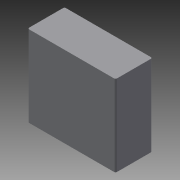
# Autodesk Inventor part: Battery(Raw)
Saved by Autodesk Inventor 2014 SP1 (Build 180222100, 222)
## iProperties
Created: 2014-03-26
Part Number: Battery(Raw)
Material: Generic
Document SubType Name: Modeling
Designer: carpenma
Density: 1 g/cm^3
Appearance: Default
Author: carpenma
Autodesk Inventor part; units mm, degrees
ref_plane "YZ Plane" through (0, 0, 0) normal (1, 0, 0) x (0, 1, 0)
ref_plane "XZ Plane" through (0, 0, 0) normal (0, 1, 0) x (-1, 0, 0)
ref_plane "XY Plane" through (0, 0, 0) normal (0, 0, 1) x (1, 0, 0)
sketch "Sketch1" plane through (0, 0, 0) normal (0, 0, 1) x (1, 0, 0)
  line L0 (0, 0) -> (181.102, 0)
  line L1 (181.102, 0) -> (181.102, 166.878)
  line L2 (181.102, 166.878) -> (0, 166.878)
  line L3 (0, 166.878) -> (0, 0)
  dimension "d0" = 181.102
  dimension "d1" = 166.878
  constraints: 8 end point, 2 parallel, 1 horizontal, 1 perpendicular
  measures "d0" distance of L2.end L1.end
  measures "d1" distance of L1.end L0.end
extrude "Extrusion1" add sketch "Sketch1" against normal blind 75.946
fillet "Fillet1" radius 3.175 4 edges at (0, 83.439, 0) (181.102, 83.439, 0) (181.102, 83.439, -75.946) (0, 83.439, -75.946)
body "Solid1"
